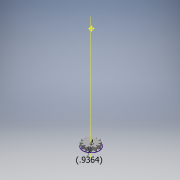
# Autodesk Inventor part: Bevel Gear2
Saved by Autodesk Inventor 2017 (Build 210142000, 142)
## iProperties
Created: 2017-01-25
Part Number: Bevel Gear2
Material: Steel, Mild
Document SubType Name: Modeling
Designer: David Kopala
Categories: <?xml version="1.0" encoding="UTF-16"?> <MemberInstance><Categories><FamilyTemplate><FamilyTemplateParameter ValueType="xs:double" Id="1" ObjectReferenceKey="da_z" ObjectType="kUserParameterObject"/><FamilyTemplateParameter ValueType="xs:double" Id="2" ObjectReferenceKey="da_b" ObjectType="kUserParameterObject"/><FamilyTemplateParameter ValueType="xs:double" Id="3" ObjectReferenceKey="da_beta" ObjectType="kUserParameterObject"/><FamilyTemplateParameter ValueType="xs:double" Id="4" ObjectReferenceKey="da_dae" ObjectType="kUserParameterObject"/><FamilyTemplateParameter ValueType="xs:double" Id="5" ObjectReferenceKey="da_ve" ObjectType="kUserParameterObject"/><FamilyTemplateParameter ValueType="xs:double" Id="6" ObjectReferenceKey="da_omega" ObjectType="kUserParameterObject"/><FamilyTemplateParameter ValueType="xs:string" Id="7" ObjectReferenceKey="EAIAABAAAAAAHwAAAAAAAIAAAAAAAAAA" ObjectType="83914240" SubObjectId="SurfaceGeometry"/></FamilyTemplate><ParamToTemplateMap><ParamToTemplate CategoryParameter="//CategoryParameter[@InternalName='046C89C9-8512-4d59-83FE-43B91F4F132A']" TemplateParameter="1"/><ParamToTemplate CategoryParameter="//CategoryParameter[@InternalName='2552DF32-E462-4b46-AEBF-C6C7768E72AC']" TemplateParameter="2"/><ParamToTemplate CategoryParameter="//CategoryParameter[@InternalName='C9EE641D-15FC-4fae-A226-E94C4372FDD7']" TemplateParameter="3"/><ParamToTemplate><ParamToTemplate CategoryParameter="//CategoryParameter[@InternalName='00B6519A-459B-49c7-AD84-2E56D39A5744']" ConstantValue="0.125000"/></ParamToTemplate><ParamToTemplate><ParamToTemplate CategoryParameter="//CategoryParameter[@InternalName='04B31F0E-C7A6-4894-AA32-9629BEFACF47']" ConstantValue="1.000000"/></ParamToTemplate><ParamToTemplate><ParamToTemplate CategoryParameter="//CategoryParameter[@InternalName='43CBEC2E-7847-49e7-A936-2F7889FCB2D9']" ConstantValue="0.200000"/></ParamToTemplate><ParamToTemplate><ParamToTemplate CategoryParameter="//CategoryParameter[@InternalName='B1EFC894-105D-4ebd-86BF-FA20ED196853']" ConstantValue="0.300000"/></ParamToTemplate><ParamToTemplate><ParamToTemplate CategoryParameter="//CategoryParameter[@InternalName='51175063-3D10-4879-93E8-6246FE8B403D']" ConstantValue="2061532430.657340"/></ParamToTemplate><ParamToTemplate><ParamToTemplate CategoryParameter="//CategoryParameter[@InternalName='A3A52E27-4454-46a9-B0BD-C932399B70AF']" ConstantValue="0.300000"/></ParamToTemplate><ParamToTemplate CategoryParameter="//CategoryParameter[@InternalName='2A200944-5A8C-41ca-B96E-8520D2E510F1']" TemplateParameter="4"/><ParamToTemplate><ParamToTemplate CategoryParameter="//CategoryParameter[@InternalName='1A637F62-92C8-44bc-B81F-10802510B579']" ConstantValue="2.297620"/></ParamToTemplate><ParamToTemplate CategoryParameter="//CategoryParameter[@InternalName='B52DD4BE-6863-48fb-BF58-89EF6F9EC65C']" TemplateParameter="5"/><ParamToTemplate><ParamToTemplate CategoryParameter="//CategoryParameter[@InternalName='3956BFF2-84D2-457d-93C2-9B0613DEBA67']" ConstantValue="14.383099"/></ParamToTemplate><ParamToTemplate CategoryParameter="//CategoryParameter[@InternalName='739CFA02-461B-4bf8-8049-181FCAD8B28F']" TemplateParameter="6"/><ParamToTemplate><ParamToTemplate CategoryParameter="//CategoryParameter[@InternalName='A27E999F-E2CE-4481-8A2A-EBF499C4C3C5']" ConstantValue="-0.000000"/></ParamToTemplate><ParamToTemplate><ParamToTemplate CategoryParameter="//CategoryParameter[@InternalName='9E1B4470-B2D3-4ff1-B813-535BB4CDF51A']" ConstantValue="3523220.976809"/></ParamToTemplate><ParamToTemplate><ParamToTemplate CategoryParameter="//CategoryParameter[@InternalName='F8452263-BFF6-458c-9FB1-07C4B99E95CD']" ConstantValue="11397033.805607"/></ParamToTemplate><ParamToTemplate><ParamToTemplate CategoryParameter="//CategoryParameter[@InternalName='3E3BB259-FD49-497f-8171-6EBC954A3479']" ConstantValue="2.000000"/></ParamToTemplate><ParamToTemplate CategoryParameter="//CategoryParameter[@InternalName='27C3BAF2-7550-4e4b-AE2C-0DB134B7D9B7']" TemplateParameter="7"/></ParamToTemplateMap><Category DisplayName="Gear" InternalName="DC85795E-93AB-48d5-8EEE-5A27447B64BD" Mnemonic="Gear"><CategoryParameter DisplayName="z" InternalName="046C89C9-8512-4d59-83FE-43B91F4F132A" Mnemonic="z"/><CategoryParameter DisplayName="b" InternalName="2552DF32-E462-4b46-AEBF-C6C7768E72AC" Mnemonic="b"/><CategoryParameter DisplayName="||b|" InternalName="C9EE641D-15FC-4fae-A226-E94C4372FDD7" Mnemonic="beta"/><CategoryParameter DisplayName="x" InternalName="00B6519A-459B-49c7-AD84-2E56D39A5744" Mnemonic="x"/><CategoryParameter DisplayName="a*" InternalName="04B31F0E-C7A6-4894-AA32-9629BEFACF47" Mnemonic="a"/><CategoryParameter DisplayName="c*" InternalName="43CBEC2E-7847-49e7-A936-2F7889FCB2D9" Mnemonic="c"/><CategoryParameter DisplayName="r|.f|*" InternalName="B1EFC894-105D-4ebd-86BF-FA20ED196853" Mnemonic="rf"/><CategoryParameter DisplayName="E" InternalName="51175063-3D10-4879-93E8-6246FE8B403D" Mnemonic="E"/><CategoryParameter DisplayName="||m|" InternalName="A3A52E27-4454-46a9-B0BD-C932399B70AF" Mnemonic="mi"/><Category DisplayName="BevelGear" InternalName="0C98F69A-0C2B-4791-B2FE-7691BB227E77" Mnemonic="BevelGear"><CategoryParameter DisplayName="d|.ae|" InternalName="2A200944-5A8C-41ca-B96E-8520D2E510F1" Mnemonic="dae"/><CategoryParameter DisplayName="d|.ai|" InternalName="1A637F62-92C8-44bc-B81F-10802510B579" Mnemonic="dai"/><CategoryParameter DisplayName="A|.e|" InternalName="B52DD4BE-6863-48fb-BF58-89EF6F9EC65C" Mnemonic="ve"/><CategoryParameter DisplayName="A|.i|" InternalName="3956BFF2-84D2-457d-93C2-9B0613DEBA67" Mnemonic="vi"/><CategoryParameter DisplayName="||S|" InternalName="739CFA02-461B-4bf8-8049-181FCAD8B28F" Mnemonic="omega"/><CategoryParameter DisplayName="x|.t|" InternalName="A27E999F-E2CE-4481-8A2A-EBF499C4C3C5" Mnemonic="xt"/><CategoryParameter DisplayName="||s||.Flim|" InternalName="9E1B4470-B2D3-4ff1-B813-535BB4CDF51A" Mnemonic="sFlim"/><CategoryParameter DisplayName="||s||.Hlim|" InternalName="F8452263-BFF6-458c-9FB1-07C4B99E95CD" Mnemonic="sHlim"/><CategoryParameter DisplayName="type" InternalName="3E3BB259-FD49-497f-8171-6EBC954A3479" Mnemonic="type"/><CategoryParameter DisplayName="PitchDiameter" InternalName="27C3BAF2-7550-4e4b-AE2C-0DB134B7D9B7" Mnemonic="IDS_PITCHDIAM"/></Category></Category></Categories></MemberInstance>
Mass: 60.9118 g
Surface Area: 34.3074 cm^2
Volume: 7.7496 cm^3
Density: 7.86 g/cm^3
Appearance: Steel
CustomPartVersion: 1
BevDriverDia: 0.9364 in
Author: David Kopala
Autodesk Inventor part; units mm, degrees
ref_plane "Mesh Plane2" through (0, 0, 0) normal (0.9659258, 0.258819, 0) x (0, 0, 1)
sketch "Teeth Body Sketch" plane through (0, 0, 0) normal (1, 0, 0) x (0, 1, 0)
  line L0 (0, 0) -> (8.3439, -149.1372) construction
  line L1 (8.3439, -149.1372) -> (11.8926, -148.8952)
  line L2 (11.8926, -148.8952) -> (0, 0) construction
  line L3 (10.16, -149.0133) -> (0, 0) construction
  line L4 (8.0601, -144.0647) -> (11.4881, -143.831)
  line L5 (8.3439, -149.1372) -> (8.0601, -144.0647)
  line L6 (11.8926, -148.8952) -> (11.4881, -143.831)
  line L7 (0, -177.9494) -> (0, 29.6582) projected
  line L8 (0, -149.0133) -> (11.8926, -149.0133) construction
  dimension "d0" = 20.32
  dimension "d1" = 16.6878
  dimension "d2" = 23.7852
  dimension "d3" = 5.08
  dimension "d4" = 148.8952
  constraints: 16 end point, 4 point on line, 3 perpendicular, 2 collinear, 1 horizontal alignment, 1 vertical alignment
  measures "d0" diameter of L3.start L7
  measures "d1" diameter of L0.end L7
  measures "d2" diameter of L1.end L7
  measures "d3" distance between parallel lines of L1 L4
  measures "d4" vertical distance of L1.end L0.start
revolve "Teeth Body" add sketch "Teeth Body Sketch" angle 360 about axis through (0, 0, 0) along (0, 0, 1)
ref_plane "Tooth Plane" through (0, 10.16, -149.0133) normal (0, -0.0680239, 0.9976837) x (1, 0, 0)
sketch "Start Sketch" plane through (0, 10.16, -149.0133) normal (0, -0.0680239, 0.9976837) x (1, 0, 0)
  line L0 (0, -12.7814) -> (0, 5.4012) projected
  arc A0 (-0.4876, -2.2472) -> (-4.1841, 2.1112) centre (-5.4662, -2.7229) ccw
  arc A1 (4.1841, 2.1112) -> (0.4876, -2.2472) centre (5.4662, -2.7229) ccw
  line L1 (-0.4876, -2.2472) -> (0.4876, -2.2472)
  arc A2 (4.1841, 2.1112) -> (-4.1841, 2.1112) centre (0, -10.1836) ccw
  dimension "d7" = 5.0013
  dimension "d8" = 5.4662
  dimension "d9" = 7.4607
  dimension "d57" = 12.9873
  dimension "d58" = 7.9364
  constraints: 6 point on circle, 3 centre point, 3 symmetric about line, 2 end point, 1 coincident, 1 perpendicular, 1 other
  measures "d7" radius of A0
  measures "d8" horizontal distance of point (0, -10.184) A0.centre
  measures "d9" vertical distance of point (0, -10.184) A0.centre
  measures "d57" radius of A2
  measures "d58" distance from line of A2.centre L1
sketch "End Sketch" plane through (0, 9.8023, -143.7677) normal (0, -0.0680239, 0.9976837) x (1, 0, 0)
  line L0 (0, -12.3315) -> (0, 5.2256) projected
  arc A0 (-0.471, -2.1601) -> (-4.041, 2.0492) centre (-5.2793, -2.6196) ccw
  arc A1 (4.041, 2.0492) -> (0.471, -2.1601) centre (5.2793, -2.6196) ccw
  line L1 (-0.471, -2.1601) -> (0.471, -2.1601)
  arc A2 (4.041, 2.0492) -> (-4.041, 2.0492) centre (0, -9.8251) ccw
  dimension "d12" = 4.8302
  dimension "d15" = 5.2793
  dimension "d16" = 7.2055
  dimension "d59" = 12.5431
  dimension "d60" = 7.665
  constraints: 6 point on circle, 3 centre point, 3 symmetric about line, 2 end point, 1 coincident, 1 other
  measures "d12" radius of A0
  measures "d15" horizontal distance of A0.centre point (0, -9.825)
  measures "d16" vertical distance of A0.centre point (0, -9.825)
  measures "d59" radius of A2
  measures "d60" distance from line of A2.centre L1
loft "Loft" cut profiles "Start Sketch", "End Sketch"
pattern_circular "Circular Pattern" count 12 over 360 about axis through (0, 0, 0) along (0, 0, 1) of "Loft"
ref_plane "End Plane" through (0, 9.8023, -143.7677) normal (0, -0.0680239, 0.9976837) x (1, 0, 0)
sketch3d "3D Sketch Right"
ref_plane "End Plane Right" through (-2.528, 9.4707, -143.7677) normal (0.0175434, -0.0657227, 0.9976837) x (0.9661714, 0.2579006, 0)
sketch "End Sketch Right" plane through (-2.528, 9.4707, -143.7677) normal (0.0175434, -0.0657227, 0.9976837) x (0.9661714, 0.2579006, 0)
  arc A0 (-0.471, -2.1601) -> (-4.041, 2.0492) centre (-5.2793, -2.6196) ccw
  line L0 (0, -16.0077) -> (0, 8.9) projected
  arc A1 (4.041, 2.0492) -> (0.471, -2.1601) centre (5.2793, -2.6196) ccw
  line L1 (-0.471, -2.1601) -> (0.471, -2.1601)
  arc A2 (4.041, 2.0492) -> (-4.041, 2.0492) centre (0, -9.8251) ccw
  dimension "d70" = 5.2793
  dimension "d71" = 7.2055
  dimension "d72" = 4.8302
  dimension "d73" = 7.665
  dimension "d74" = 12.5431
  constraints: 6 point on circle, 3 centre point, 3 symmetric about line, 2 end point, 1 coincident, 1 perpendicular, 1 other
  measures "d70" horizontal distance of A2.centre A0.centre
  measures "d71" vertical distance of point (0, -9.825) A0.centre
  measures "d72" radius of A0
  measures "d73" distance from line of point (0, -9.825) L1
  measures "d74" radius of A2
feature "Loft Right" [suppressed]
pattern_circular "Circular Pattern Right" [suppressed]
sketch3d "3D Sketch Left"
ref_plane "End Plane Left" through (2.5204, 9.4707, -143.764) normal (-0.0174912, -0.0657245, 0.9976845) x (0.966364, -0.2571783, 0)
sketch "End Sketch Left" plane through (2.5204, 9.4707, -143.764) normal (-0.0174912, -0.0657245, 0.9976845) x (0.966364, -0.2571783, 0)
  line L0 (0, -34.0046) -> (0, 15.4849) projected
  arc A0 (-0.471, -2.1584) -> (-4.041, 2.0509) centre (-5.2793, -2.6179) ccw
  arc A1 (4.041, 2.0509) -> (0.471, -2.1584) centre (5.2793, -2.6179) ccw
  line L1 (-0.471, -2.1584) -> (0.471, -2.1584)
  ellipse E0 centre (0, -9.7822) end of major axis (11.4881, -9.7822) minor radius 11.4615 projected
  arc A2 (4.041, 2.0509) -> (-4.041, 2.0509) centre (0, -9.8234) ccw
  dimension "d56" = 11.4615
  dimension "d30" = 4.8302
  dimension "d31" = 5.2793
  dimension "d32" = 7.2055
  dimension "d61" = 12.5431
  dimension "d62" = 7.665
  constraints: 6 point on circle, 3 centre point, 3 symmetric about line, 2 end point, 1 coincident, 2 other
  measures "d30" radius of A0
  measures "d31" horizontal distance of point (0, -9.823) A0.centre
  measures "d32" vertical distance of A0.centre point (0, -9.823)
  measures "d61" radius of A2
  measures "d62" distance from line of point (0, -9.823) L1
feature "Loft Left" [suppressed]
pattern_circular "Circular Pattern Left" [suppressed]
sketch "Body Sketch" plane through (0, 0, 0) normal (1, 0, 0) x (0, 1, 0)
  line L0 (0, -149.3057) -> (0, -142.2044) projected
  line L1 (8.3439, -149.1372) -> (8.0601, -144.0647) projected
  line L2 (8.0601, -144.0647) -> (0, -144.0647)
  line L3 (8.3439, -149.1372) -> (0, -149.1372)
  constraints: 4 end point, 2 perpendicular, 2 point on line
revolve "Fix Body" add sketch "Body Sketch" angle 360 about axis through (0, 0, 0) along (0, 0, 1)
sketch "Sketch6" plane through (0, 0, 0) normal (1, 0, 0) x (0, 1, 0)
  line L0 (10.16, -149.0133) -> (0, 0) projected
  line L1 (0, -177.8) -> (0, 29.6333) projected
surface revolve "Pitch Diameter" sketch "Sketch6" angle 360 about axis through (0, 0, 0) along (0, 0, 1) shown no curves L0
sketch "Sketch8" plane through (0, 0, -149.1372) normal (0, 0, -1) x (-1, 0, 0)
  circle A0 centre (0, 0) radius 11.8926
  arc A1 (-8.6936, -8.1151) -> (-8.1151, -8.6936) centre (0, 0) ccw projected
  dimension "BevDriverDia" = 23.7852
  constraints: 1 centre point, 1 coincident, 1 concentric
  measures "BevDriverDia" diameter of A0
equation "\"d0\" = da_de"
equation "\"d1\" = da_dfe"
equation "\"d2\" = da_dae"
equation "\"d3\" = da_b"
equation "\"d4\" = da_ve"
equation "\"d7\" = fd_rr"
equation "\"d8\" = fd_x"
equation "\"d9\" = fd_y"
equation "\"d57\" = 0.5 * fd_dva + 0.3 * da_he"
equation "\"d58\" = 0.5 * fd_dva - 1.12 * da_he"
equation "\"da_teethtype\" = 0"
equation "\"da_b\" = 5.08"
equation "\"da_de\" = 20.32"
equation "\"da_dae\" = 23.78518"
equation "\"da_dfe\" = 16.68777"
equation "\"da_le\" = 149.3593"
equation "\"da_omega\" = 90deg"
equation "\"da_beta\" = 0"
equation "\"da_delta\" = 3.900494deg"
equation "\"da_alpha\" = 25deg"
equation "\"da_he\" = 3.55694"
equation "\"da_ve\" = 148.8952"
equation "\"da_zv\" = 12.02786"
equation "\"fd_loft\" = da_b + 0.05 * da_he"
equation "\"fd_x\" = fd_x1 + fd_x2"
equation "\"fd_y\" = fd_y1 - fd_y2"
equation "\"fd_dd\" = fd_dva - 0.8 * da_he"
equation "\"da_dvw\" = 20.79051"
equation "\"d11\" = fd_loft"
equation "\"da_dm\" = 19.97444"
equation "\"da_x\" = 0.125"
equation "\"da_m\" = 1.69333"
equation "\"d50\" = da_omega"
equation "\"fd_rr\" = 5.001282"
equation "\"fd_dva\" = 23.840397"
equation "\"fd_x1\" = 1.353728"
equation "\"fd_x2\" = 4.112514"
equation "\"fd_y1\" = 10.306733"
equation "\"fd_y2\" = 2.846058"
body "Solid1"
body "Srf1"
